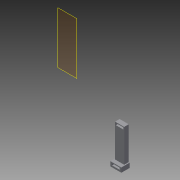
# Autodesk Inventor part: side piece
Saved by Autodesk Inventor 2015 (Build 190159000, 159)
## iProperties
Created: 2014-11-22
Part Number: side piece
Material: Generic
Document SubType Name: Modeling
Designer: jesse
Density: 1 g/cm^3
Appearance: Default
d2: 0.500 in
d3: 0.00 deg
d4: 0.100 in
d5: 0.00 deg
d6: 0.125 in
d9: 0.125 in
d10: 0.125 in
d11: 0.125 in
d13: 0.00 deg
d14: 0.500 in
d15: 0.00 deg
d16: 0.750 in
d17: 0.200 in
d18: 0.200 in
d19: 0.500 in
d20: 0.00 deg
d22: 0.00 deg
d23: 0.875 in
d24: 0.125 in
d25: 0.125 in
d27: 0.00 deg
Author: jesse
Autodesk Inventor part; units mm, degrees
ref_plane "YZ Plane" through (0, 0, 0) normal (1, 0, 0) x (0, 1, 0)
ref_plane "XZ Plane" through (0, 0, 0) normal (0, 1, 0) x (-1, 0, 0)
ref_plane "XY Plane" through (0, 0, 0) normal (0, 0, 1) x (1, 0, 0)
ref_plane "Work Plane1" through (29.6407, 50.9726, 24.365) normal (0, 0, -1) x (-1, 0, 0)
sketch "Sketch1" plane through (29.6407, 50.9726, 24.365) normal (0, 0, -1) x (-1, 0, 0)
  line L0 (12.7, 3.175) -> (-12.7, 3.175) projected
  line L1 (-12.7, 3.175) -> (-12.7, -3.175) projected
  line L2 (-12.7, -3.175) -> (12.7, -3.175) projected
  line L3 (12.7, -3.175) -> (12.7, 3.175) projected
  line L4 (-12.7, -113.4117) -> (12.7, -113.4117) projected
  line L5 (12.7, -113.4117) -> (12.7, -107.0617) projected
  line L6 (12.7, -107.0617) -> (-12.7, -107.0617) projected
  line L7 (-12.7, -107.0617) -> (-12.7, -113.4117) projected
  line L8 (-15.24, -5.715) -> (-15.24, 5.715)
  line L9 (-15.24, 5.715) -> (15.24, 5.715)
  line L10 (15.24, 5.715) -> (15.24, -5.715)
  line L11 (15.24, -96.743) -> (15.24, -115.9518)
  line L12 (15.24, -115.9518) -> (-15.24, -115.9518)
  line L13 (-15.24, -115.9518) -> (-15.24, -96.743)
  line L14 (-15.24, -5.715) -> (-15.24, -96.743)
  line L15 (15.24, -5.715) -> (15.24, -98.1393)
  point P0 (29.6407, -50.9726)
  constraints: 16 end point, 1 point on line, 4 other
extrude "Extrusion1" add sketch "Sketch1" against normal blind 12.7
sketch "Sketch2" plane through (29.6407, 50.9726, 24.365) normal (0, 0, -1) x (-1, 0, 0)
  line L0 (15.24, -115.9518) -> (15.24, 5.715) projected
  line L1 (-15.24, -115.9518) -> (15.24, -115.9518) projected
  line L2 (-15.24, 5.715) -> (-15.24, -115.9518) projected
  line L3 (15.24, 5.715) -> (-15.24, 5.715) projected
  point P0 (29.6407, -50.9726)
extrude "Extrusion2" add sketch "Sketch2" along normal blind 2.54
sketch "Sketch3" plane through (29.6407, 50.9726, 37.065) normal (0, 0, 1) x (1, 0, 0)
  line L0 (-12.7, -113.4117) -> (-12.7, -107.0617) projected
  line L1 (-12.7, -107.0617) -> (12.7, -107.0617) projected
  line L2 (12.7, -107.0617) -> (12.7, -113.4117) projected
  line L3 (12.7, -113.4117) -> (-12.7, -113.4117) projected
  line L4 (12.7, 3.175) -> (12.7, -3.175) construction
  line L5 (12.7, -3.175) -> (-12.7, -3.175) construction
  line L6 (-12.7, -3.175) -> (-12.7, 3.175) construction
  line L7 (-12.7, 3.175) -> (12.7, 3.175) construction
  line L8 (-15.24, 5.715) -> (-15.24, -115.9518) construction
  line L9 (-15.24, -115.9518) -> (15.24, -115.9518) construction
  line L10 (15.24, -115.9518) -> (15.24, 5.715) construction
  line L11 (15.24, 5.715) -> (-15.24, 5.715) construction
  line L12 (18.415, -119.1268) -> (-18.415, -119.1268)
  line L13 (-18.415, -119.1268) -> (-18.415, -103.8867)
  line L14 (-18.415, -103.8867) -> (18.415, -103.8867)
  line L15 (18.415, -103.8867) -> (18.415, -119.1268)
  line L16 (18.415, -119.1268) -> (-18.415, -103.8867) construction
  line L17 (-18.415, -119.1268) -> (18.415, -103.8867) construction
  point P0 (-29.6407, -50.9726)
  point P1 (0, -111.5068)
  dimension "d6" = 3.175
  dimension "d9" = 3.175
  dimension "d10" = 3.175
  dimension "d11" = 3.175
  constraints: 12 end point, 2 midpoint, 2 parallel, 1 horizontal, 1 perpendicular
  measures "d6" distance between parallel lines of L12 L9
  measures "d9" distance between parallel lines of L15 L10
  measures "d10" distance between parallel lines of L13 L8
  measures "d11" distance between parallel lines of L1 L14
extrude "Extrusion3" add sketch "Sketch3" against normal up to surface (15.24 mm away)
sketch "Sketch4" plane through (29.6407, 50.9726, 37.065) normal (0, 0, 1) x (1, 0, 0)
  line L0 (-12.7, -113.4117) -> (-12.7, -107.0617) projected
  line L1 (-12.7, -107.0617) -> (12.7, -107.0617) projected
  line L2 (12.7, -107.0617) -> (12.7, -113.4117) projected
  line L3 (12.7, -113.4117) -> (-12.7, -113.4117) projected
  line L4 (-18.415, -103.8867) -> (-15.24, -103.8867) projected
  line L5 (-18.415, -119.1268) -> (-18.415, -103.8867) projected
  line L6 (18.415, -119.1268) -> (-18.415, -119.1268) projected
  line L7 (18.415, -103.8867) -> (18.415, -119.1268) projected
  line L8 (15.24, -103.8867) -> (18.415, -103.8867) projected
  line L9 (15.24, -103.8867) -> (15.24, 5.715) projected
  line L10 (15.24, 5.715) -> (-15.24, 5.715) projected
  line L11 (-15.24, 5.715) -> (-15.24, -103.8867) projected
  line L12 (12.7, 3.175) -> (12.7, -3.175) projected
  line L13 (12.7, -3.175) -> (-12.7, -3.175) projected
  line L14 (-12.7, -3.175) -> (-12.7, 3.175) projected
  line L15 (-12.7, 3.175) -> (12.7, 3.175) projected
  line L16 (15.24, -103.8867) -> (-15.24, -103.8867)
  point P0 (-29.6407, -50.9726)
  constraints: 2 end point, 1 horizontal
extrude "Extrusion4" add sketch "Sketch4" along normal blind 12.7 contours L4 L16 L8 L7 L6 L5
sketch "Sketch5" plane through (29.6407, 50.9726, 37.065) normal (0, 0, 1) x (1, 0, 0)
  line L0 (-15.24, -103.8867) -> (-15.24, 5.715) projected
  line L1 (-15.24, 5.715) -> (15.24, 5.715) projected
  line L2 (15.24, 5.715) -> (15.24, -103.8867) projected
  line L3 (18.415, -103.8867) -> (15.24, -103.8867) projected
  line L4 (18.415, -119.1268) -> (18.415, -103.8867) projected
  line L5 (-18.415, -119.1268) -> (18.415, -119.1268) projected
  line L6 (-18.415, -103.8867) -> (-18.415, -119.1268) projected
  line L7 (-15.24, -103.8867) -> (-18.415, -103.8867) projected
  line L8 (15.24, -103.8867) -> (15.24, 5.715) construction
  line L9 (15.24, -49.0859) -> (-15.24, -49.0859) construction
  line L10 (-15.24, 5.715) -> (-15.24, -103.8867) construction
  line L11 (0, -49.0859) -> (0, -119.1268) construction
  line L12 (-18.415, -119.1268) -> (18.415, -119.1268) construction
  line L13 (0, -49.0859) -> (0, 5.715) construction
  line L14 (15.24, 5.715) -> (-15.24, 5.715) construction
  line L15 (-15.24, -39.5609) -> (15.24, -39.5609)
  line L16 (15.24, -39.5609) -> (15.24, -58.6109)
  line L17 (15.24, -58.6109) -> (-15.24, -58.6109)
  line L18 (-15.24, -58.6109) -> (-15.24, -39.5609)
  line L19 (-15.24, -39.5609) -> (15.24, -58.6109) construction
  line L20 (15.24, -39.5609) -> (-15.24, -58.6109) construction
  line L21 (15.24, -39.5609) -> (-15.24, -39.5609)
  line L22 (-15.24, -39.5609) -> (-15.24, -34.4809)
  line L23 (-15.24, -34.4809) -> (15.24, -34.4809)
  line L24 (15.24, -34.4809) -> (15.24, -39.5609)
  line L25 (15.24, -58.6109) -> (-15.24, -58.6109)
  line L26 (-15.24, -58.6109) -> (-15.24, -63.6909)
  line L27 (-15.24, -63.6909) -> (15.24, -63.6909)
  line L28 (15.24, -63.6909) -> (15.24, -58.6109)
  point P0 (-29.6407, -50.9726)
  dimension "d16" = 19.05
  dimension "d17" = 5.08
  dimension "d18" = 5.08
  constraints: 34 end point, 7 midpoint, 6 parallel, 3 horizontal, 3 perpendicular, 3 point on line
  measures "d16" distance of L15.end L16.end
  measures "d17" distance between parallel lines of L21 L23
  measures "d18" distance between parallel lines of L25 L27
extrude "Extrusion5" add sketch "Sketch5" along normal blind 12.7 contours L0 L17 L2 L27 | L0 L23 L2 L15
sketch "Sketch6" plane through (14.4007, 56.6876, 21.825) normal (-1, 0, 0) x (0, 0, 1)
  line L0 (0, -109.6018) -> (15.24, -109.6018) projected
  line L1 (15.24, -69.4059) -> (15.24, -109.6018) projected
  line L2 (15.24, -69.4059) -> (27.94, -69.4059) projected
  line L3 (27.94, -64.3259) -> (27.94, -69.4059) projected
  line L4 (15.24, -64.3259) -> (27.94, -64.3259) projected
  line L5 (15.24, -45.2759) -> (15.24, -64.3259) projected
  line L6 (15.24, -45.2759) -> (27.94, -45.2759) projected
  line L7 (27.94, -40.1959) -> (27.94, -45.2759) projected
  line L8 (15.24, -40.1959) -> (27.94, -40.1959) projected
  line L9 (15.24, 0) -> (15.24, -40.1959) projected
  line L10 (15.24, 0) -> (0, 0) projected
  line L11 (0, -109.6018) -> (0, 0) projected
  line L12 (15.24, -40.1959) -> (27.94, -45.2759)
  line L13 (27.94, -64.3259) -> (15.24, -69.4059)
  point P0 (-21.825, -56.6876)
  constraints: 4 end point
extrude "Extrusion6" cut sketch "Sketch6" against normal through all contours L13 L3 L2 | L8 L7 L12
fillet "Fillet1" radius 22.225 2 edges at (29.6407, -12.7183, 37.065) (29.6407, 16.4917, 37.065)
sketch "Sketch7" plane through (29.6407, 50.9726, 37.065) normal (0, 0, 1) x (1, 0, 0)
  line L0 (15.24, -39.5609) -> (-15.24, -39.5609) projected
  line L1 (-15.24, -39.5609) -> (-15.24, -58.6109) projected
  line L2 (-15.24, -58.6109) -> (15.24, -58.6109) projected
  line L3 (15.24, -58.6109) -> (15.24, -39.5609) projected
  line L4 (-15.24, -49.0859) -> (15.24, -49.0859) construction
  line L5 (0, -58.6109) -> (0, -39.5609) construction
  circle A0 centre (-8.1605, -49.0859) radius 1.5875
  circle A1 centre (8.1605, -49.0859) radius 1.5875
  line L6 (-8.1605, -49.0859) -> (-8.1605, -44.6177) construction
  line L7 (8.1605, -49.0859) -> (8.1605, -44.6177) construction
  line L8 (8.1605, -44.8596) -> (0, -44.8596) construction
  line L9 (0, -44.8596) -> (-8.1605, -44.8596) construction
  point P0 (-29.6407, -50.9726)
  dimension "d24" = 3.175
  dimension "d25" = 3.175
  constraints: 12 end point, 6 point on line, 4 midpoint, 2 centre point, 2 vertical, 1 collinear, 1 perpendicular
  measures "d24" diameter of A0
  measures "d25" diameter of A1
extrude "Extrusion7" cut sketch "Sketch7" against normal through all contours A0 | A1
body "Solid1"
